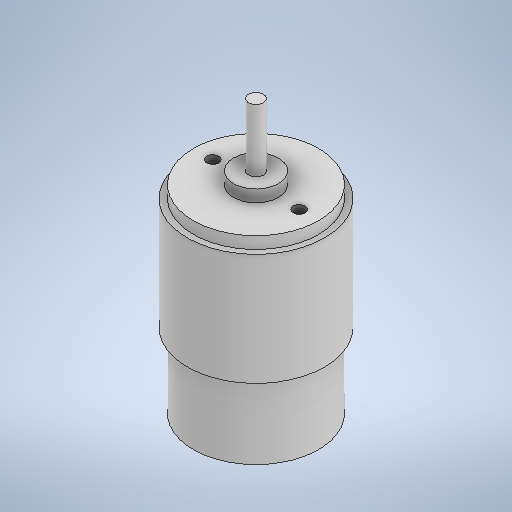
# Autodesk Inventor part: motor
Saved by Autodesk Inventor 2025 (Build 290162000, 162)
## iProperties
Created: 2025-04-03
Part Number: motor
Material: 일반
Document SubType Name: Modeling
Designer: 112-ROBOT-10
Density: 1 g/cm^3
Appearance: 기본값
Author: 112-ROBOT-10
Autodesk Inventor part; units mm, degrees
ref_plane "YZ Plane" through (0, 0, 0) normal (1, 0, 0) x (0, 1, 0)
ref_plane "XZ Plane" through (0, 0, 0) normal (0, 1, 0) x (-1, 0, 0)
sketch "스케치1" plane through (0, 0, 0) normal (0, 1, 0) x (-1, 0, 0)
  circle A0 centre (0, 0) radius 21
  dimension "d0" = 42
  constraints: 1 centre point, 1 coincident
  measures "d0" diameter of A0
extrude "돌출1" add sketch "스케치1" along normal blind 66.5
sketch "스케치2" plane through (0, 66.5, 0) normal (0, 1, 0) x (1, 0, 0)
  circle A0 centre (0, 0) radius 7.5
  dimension "d3" = 15
  constraints: 1 centre point, 1 coincident
  measures "d3" diameter of A0
extrude "돌출2" add sketch "스케치2" along normal blind 4
sketch "스케치3" plane through (0, 70.5, 0) normal (0, 1, 0) x (1, 0, 0)
  circle A0 centre (0, 0) radius 2.5
  dimension "d6" = 5
  constraints: 1 centre point, 1 coincident
  measures "d6" diameter of A0
extrude "돌출3" add sketch "스케치3" along normal blind 21
sketch "스케치4" plane through (0, 66.5, 0) normal (0, 1, 0) x (1, 0, 0)
  circle A0 centre (-14.5, 0) radius 2
  circle A1 centre (14.5, 0) radius 2
  line L0 (-14.5, 0) -> (14.5, 0)
  point P0 (0, 0)
  point P1 (0, 0)
  dimension "d9" = 4
  dimension "d10" = 4
  dimension "d11" = 29
  constraints: 2 centre point, 2 end point, 2 horizontal alignment, 1 coincident, 1 horizontal, 1 midpoint
  measures "d9" diameter of A0
  measures "d10" diameter of A1
  measures "d11" distance of L0.end L0.start
extrude "돌출4" cut sketch "스케치4" against normal blind 15
thread "스레드1" size "M4x0.7" class "6H" standard "ANSI Metric M Profile" full length
thread "스레드2" size "M4x0.7" class "6H" standard "ANSI Metric M Profile" full length
ref_plane "작업 평면1" through (0, 62.5, 0) normal (0, 1, 0) x (1, 0, 0)
sketch "스케치5" plane through (0, 62.5, 0) normal (0, 1, 0) x (1, 0, 0)
  circle A0 centre (0, 0) radius 2.5 projected
  circle A1 centre (0, 0) radius 23
  dimension "d19" = 46
  constraints: 1 centre point, 1 coincident
  measures "d19" diameter of A1
extrude "돌출5" add sketch "스케치5" against normal blind 37.5
